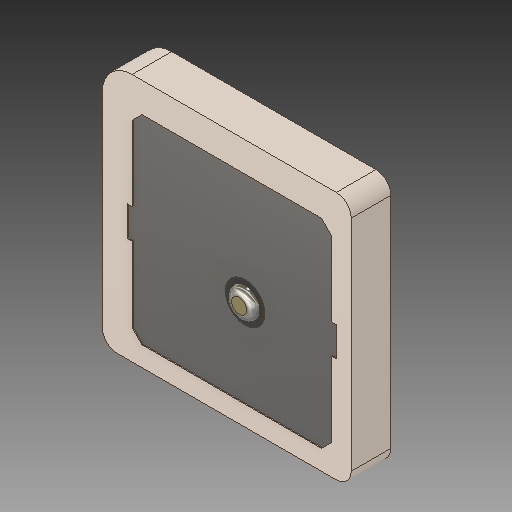
# Autodesk Inventor part: Antenna_GPSPatch
Saved by Autodesk Inventor 2018 (Build 220112000, 112)
## iProperties
Created: 2018-01-04
Part Number: Antenna_GPSPatch
Material: Porcelain, Linen
Document SubType Name: Modeling
Designer: Bradley
Density: 3.4 g/cm^3
Appearance: Sandy Taupe
Stock Number: GP.1575.25.4.A.02
Author: Bradley
Autodesk Inventor part; units mm, degrees
ref_plane "XZ Plane" through (0, 0, 0) normal (0, 1, 0) x (-1, 0, 0)
ref_plane "XY Plane" through (0, 0, 0) normal (0, 0, 1) x (1, 0, 0)
sketch "Sketch1" plane through (0, 0, 0) normal (0, 0, 1) x (1, 0, 0)
  line L0 (-11.05, -12.55) -> (11.05, -12.55)
  line L1 (12.55, -11.05) -> (12.55, 11.05)
  line L2 (11.05, 12.55) -> (-9.55, 12.55)
  line L3 (-12.55, 9.55) -> (-12.55, -11.05)
  line L4 (-12.55, -12.55) -> (12.55, 12.55) construction
  line L5 (12.55, -12.55) -> (-12.55, 12.55) construction
  arc A0 (-9.55, 12.55) -> (-12.55, 9.55) centre (-9.55, 9.55) ccw
  arc A1 (-12.55, -11.05) -> (-11.05, -12.55) centre (-11.05, -11.05) ccw
  arc A2 (11.05, -12.55) -> (12.55, -11.05) centre (11.05, -11.05) ccw
  arc A3 (12.55, 11.05) -> (11.05, 12.55) centre (11.05, 11.05) ccw
  circle A4 centre (1.75, -1.75) radius 0.45
  point P0 (0, 0)
  point P1 (0, 0)
  dimension "d0" = 25.1
  dimension "d1" = 3
  dimension "d2" = 0.9
  dimension "d7" = 1.5
  dimension "d8" = 25.1
  dimension "d9" = 1.75
  constraints: 12 end point, 9 point on line, 8 point on circle, 8 tangent, 5 centre point, 3 midpoint, 2 equal radius, 2 parallel, 1 horizontal, 1 perpendicular
  measures "d0" distance of L5.end L4.end
  measures "d1" radius of A0
  measures "d2" diameter of A4
  measures "d7" radius of A3
  measures "d8" distance between parallel lines of L0 L2
  measures "d9" horizontal distance of A4.centre point (0, 0)
extrude "Extrusion1" add sketch "Sketch1" along normal mid plane 4 contours A1 L3 A0 L2 A3 L1 A2 L0 | A4
extrude "Extrusion2" add sketch "Sketch1" against normal blind 4.4 and the other way blind 2.25 contours A4
chamfer "Chamfer1" distance 0.1 angle 45 1 edges at (1.3, -1.75, -4.4)
sketch "Sketch4" plane through (0, 0, 2) normal (0, 0, 1) x (1, 0, 0)
  line L0 (-12.55, 9.55) -> (-12.55, -11.05) projected
  arc A0 (-12.55, -11.05) -> (-11.05, -12.55) centre (-11.05, -11.05) ccw projected
  line L1 (-11.05, -12.55) -> (11.05, -12.55) projected
  arc A1 (11.05, -12.55) -> (12.55, -11.05) centre (11.05, -11.05) ccw projected
  line L2 (12.55, -11.05) -> (12.55, 11.05) projected
  arc A2 (12.55, 11.05) -> (11.05, 12.55) centre (11.05, 11.05) ccw projected
  line L3 (11.05, 12.55) -> (-9.55, 12.55) projected
  arc A3 (-9.55, 12.55) -> (-12.55, 9.55) centre (-9.55, 9.55) ccw projected
  line L4 (-8.55, 9.55) -> (9.55, 9.55)
  line L5 (10.55, 8.55) -> (10.55, -9.55)
  line L6 (9.55, -10.55) -> (-8.55, -10.55)
  line L7 (-9.55, -9.55) -> (-9.55, 8.55)
  line L8 (-8.55, 9.55) -> (-9.55, 8.55)
  line L9 (9.55, 9.55) -> (10.55, 8.55)
  line L10 (10.55, -9.55) -> (9.55, -10.55)
  line L11 (-8.55, -10.55) -> (-9.55, -9.55)
  line L12 (-9.55, 1) -> (-10.05, 1)
  line L13 (-10.05, 1) -> (-10.05, -2)
  line L14 (-10.05, -2) -> (-9.55, -2)
  line L15 (-9.55, -2) -> (-9.55, 1)
  line L16 (10.55, 1) -> (11.05, 1)
  line L17 (11.05, 1) -> (11.05, -2)
  line L18 (11.05, -2) -> (10.55, -2)
  line L19 (10.55, -2) -> (10.55, 1)
  point P0 (0, 0)
  point P1 (10.55, -10.55)
  point P2 (10.55, 9.55)
  point P3 (-9.55, -10.55)
  point P4 (10.55, -0.5)
  point P5 (-9.55, -0.5)
  dimension "d21" = 1
  dimension "d22" = 1
  dimension "d23" = 1
  dimension "d24" = 1
  dimension "d25" = 1
  dimension "d26" = 1
  dimension "d27" = 1
  dimension "d28" = 1
  dimension "d29" = 2
  dimension "d30" = 2
  dimension "d31" = 3
  dimension "d32" = 3
  dimension "d33" = 0.5
  dimension "d34" = 3
  constraints: 32 end point, 11 point on line, 6 parallel, 4 midpoint, 3 horizontal, 3 perpendicular, 1 collinear
  measures "d21" distance of L4.start point (-9.55, 9.55)
  measures "d22" distance of L7.end point (-9.55, 9.55)
  measures "d23" distance of L4.end point (10.55, 9.55)
  measures "d24" distance of L5.start point (10.55, 9.55)
  measures "d25" distance of L5.end point (10.55, -10.55)
  measures "d26" distance of L6.start point (10.55, -10.55)
  measures "d27" distance of L6.end point (-9.55, -10.55)
  measures "d28" distance of L7.start point (-9.55, -10.55)
  measures "d29" distance between parallel lines of L2 L5
  measures "d30" distance between parallel lines of L1 L6
  measures "d31" distance between parallel lines of L0 L7
  measures "d32" distance between parallel lines of L3 L4
  measures "d33" distance between parallel lines of L19 L17
  measures "d34" distance of L16.end L17.end
extrude "Extrusion3" cut sketch "Sketch4" against normal blind 0.1 contours L4 L9 L5 L10 L6 L11 L7 L8 | L7 L14 L13 L12 | L16 L17 L18 L5
ref_plane "Work Plane1" through (1.75, -1.75, 0) normal (1, 0, 0) x (0, 1, 0)
sketch "Sketch5" plane through (1.75, -1.75, 0) normal (1, 0, 0) x (0, 1, 0)
  line L0 (10.3, 1.9) -> (2.75, 1.9) projected
  line L1 (11.3, 1.9) -> (10.3, 1.9) projected
  line L2 (10.3, 1.9) -> (11.3, 1.9) projected
  line L3 (2.75, 1.9) -> (10.3, 1.9) projected
  line L4 (-0.25, 1.9) -> (2.75, 1.9) projected
  line L5 (-7.8, 1.9) -> (-0.25, 1.9) projected
  line L6 (-8.8, 1.9) -> (-7.8, 1.9) projected
  line L7 (-7.8, 1.9) -> (-8.8, 1.9) projected
  line L8 (-0.25, 1.9) -> (-7.8, 1.9) projected
  line L9 (2.75, 1.9) -> (-0.25, 1.9) projected
  arc A0 (-0.75, 2.5) -> (-1.5, 1.9) centre (-0.75, 1.7312) ccw
  arc A1 (1.5, 1.9) -> (0.75, 2.5) centre (0.75, 1.7312) ccw
  line L10 (-0.75, 2.5) -> (0.75, 2.5)
  line L11 (0.45, -2) -> (-0.45, -2) projected
  line L12 (-0.45, -4.3) -> (0.45, -4.3) projected
  line L13 (0, 2.5) -> (0, 1.9)
  point P0 (1.75, 0)
  point P1 (0, -2)
  dimension "d37" = 1.5
  dimension "d38" = 3
  dimension "d39" = 0.6
  constraints: 4 end point, 4 point on circle, 3 point on line, 2 centre point, 2 midpoint, 2 tangent, 1 equal radius, 1 horizontal, 1 perpendicular, 1 vertical alignment
  measures "d37" distance of L10.start L10.end
  measures "d38" distance of A1.start A0.end
  measures "d39" distance between parallel lines of L8 L10
revolve "Revolution2" add sketch "Sketch5" angle 360 about axis through (1.75, -1.75, 2.5) along (0, 0, -1) contours L13 L10 A1 L4
sketch "Sketch6" plane through (0, 0, 1.9) normal (0, 0, 1) x (1, 0, 0)
  circle A0 centre (1.75, -1.75) radius 1.5 projected
  line L0 (10.55, 1) -> (11.05, 1) projected
  line L1 (10.55, 8.55) -> (10.55, 1) projected
  line L2 (9.55, 9.55) -> (10.55, 8.55) projected
  line L3 (-8.55, 9.55) -> (9.55, 9.55) projected
  line L4 (-9.55, 8.55) -> (-8.55, 9.55) projected
  line L5 (-9.55, 1) -> (-9.55, 8.55) projected
  line L6 (-10.05, 1) -> (-9.55, 1) projected
  line L7 (-10.05, -2) -> (-10.05, 1) projected
  line L8 (-9.55, -2) -> (-10.05, -2) projected
  line L9 (-9.55, -9.55) -> (-9.55, -2) projected
  line L10 (-8.55, -10.55) -> (-9.55, -9.55) projected
  line L11 (9.55, -10.55) -> (-8.55, -10.55) projected
  line L12 (10.55, -9.55) -> (9.55, -10.55) projected
  line L13 (10.55, -2) -> (10.55, -9.55) projected
  line L14 (11.05, -2) -> (10.55, -2) projected
  line L15 (11.05, 1) -> (11.05, -2) projected
  circle A1 centre (1.75, -1.75) radius 2
  point P0 (0, 0)
  dimension "d41" = 4
  constraints: 1 centre point, 1 coincident
  measures "d41" diameter of A1
split_face "Split1"
equation "\"d8\" = d0"
equation "\"d22\" = d21"
equation "\"d23\" = d21"
equation "\"d24\" = d23"
equation "\"d25\" = d21"
equation "\"d26\" = d25"
equation "\"d27\" = d21"
equation "\"d28\" = d27"
equation "\"d30\" = d29"
body "Solid1"
